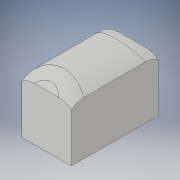
# Autodesk Inventor part: LEDS1
Saved by Autodesk Inventor 2019 (Build 230136000, 136)
## iProperties
Created: 2018-12-21
Part Number: LEDS1
Material: Типовые
Document SubType Name: Modeling
Designer: aldanstar
Density: 1 g/cm^3
Appearance: По умолчанию
Author: aldanstar
Autodesk Inventor part; units mm, degrees
ref_plane "YZ Plane" through (0, 0, 0) normal (1, 0, 0) x (0, 1, 0)
ref_plane "XZ Plane" through (0, 0, 0) normal (0, 1, 0) x (-1, 0, 0)
ref_plane "XY Plane" through (0, 0, 0) normal (0, 0, 1) x (1, 0, 0)
sketch "Эскиз1" plane through (0, 0, 0) normal (0, 1, 0) x (-1, 0, 0)
  line L0 (-1.4, -2.45) -> (1.4, -2.45)
  line L1 (1.4, -2.45) -> (1.4, 2.45)
  line L2 (1.4, 2.45) -> (-1.4, 2.45)
  line L3 (-1.4, 2.45) -> (-1.4, -2.45)
  line L4 (0, -2.45) -> (0, 2.45) construction
  line L5 (0, -3.43) -> (0, 3.43) projected
  line L6 (1.96, 0) -> (-1.96, 0) projected
  point P0 (0, 0)
  dimension "d0" = 4.9
  dimension "d2" = 2.8
  constraints: 10 end point, 2 midpoint, 2 parallel, 1 horizontal, 1 perpendicular, 2 other
  measures "d0" distance of L0.end L1.end
  measures "d2" distance between parallel lines of L1 L3
extrude "Выдавливание1" add sketch "Эскиз1" along normal blind 4
chamfer "Фаска1" distance 1 angle 45 4 edges at (0, 4, 2.45) (1.4, 4, 0) (-1.4, 4, 0) (0, 4, -2.45)
fillet "Сопряжение1" radius 2 4 edges at (0.4, 4, 0) (0, 4, 1.45) (-0.4, 4, 0) (0, 4, -1.45)
fillet "Сопряжение2" radius 1 10 edges at (1.3999, 2.9999, 2.45) (1.1083, 3.2364, 2.2136) (-1.1083, 3.2364, 2.2136) (-1.3999, 2.9999, 2.45) (0.0006, 3.5716, 1.8586) (-1.3999, 2.9999, -2.45) (-1.1083, 3.2364, -2.2136) (1.3999, 2.9999, -2.45) (1.1083, 3.2364, -2.2136) (0.0006, 3.5716, -1.8586)
